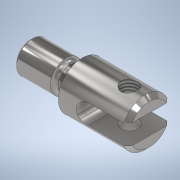
# Autodesk Inventor part: Part11.End Fork
Saved by Autodesk Inventor 2022.2 (Build 262287010, 287A)
## iProperties
Created: 2022-12-06
Part Number: Part11.End Fork
Material: Steel, Carbon
Document SubType Name: Modeling
Designer: User
Density: 7.85 g/cm^3
Appearance: Steel - Polished
Author: User
Autodesk Inventor part; units mm, degrees
ref_plane "YZ Plane" through (0, 0, 0) normal (1, 0, 0) x (0, 1, 0)
ref_plane "XY Plane" through (0, 0, 0) normal (0, 0, 1) x (1, 0, 0)
sketch "Sketch1" plane through (0, 0, 0) normal (1, 0, 0) x (0, 1, 0)
  circle A0 centre (0, 0) radius 12
  dimension "d0" = 24
  constraints: 1 centre point, 1 coincident
  measures "d0" diameter of A0
extrude "Extrusion1" add sketch "Sketch1" along normal blind 34
chamfer "Chamfer1" distance 2 angle 45 1 edges at (34, -12, 0)
sketch "Sketch2" plane through (0, 0, 0) normal (0, 0, 1) x (1, 0, 0)
  line L0 (0, -12) -> (0, 12) construction
  line L1 (32, -12) -> (32, 12) construction
  line L2 (0, 0) -> (32, 0) construction
  line L3 (14, 5) -> (34, 5)
  line L4 (34, -5) -> (14, -5)
  line L5 (34, 10) -> (34, -10) projected
  arc A0 (14, 5) -> (14, -5) centre (14, 0) ccw
  dimension "d8" = 10
  dimension "d9" = 5
  constraints: 6 end point, 2 point on circle, 2 tangent, 1 centre point, 1 horizontal, 1 midpoint, 1 parallel
  measures "d8" distance between parallel lines of L4 L3
  measures "d9" radius of A0
extrude "Extrusion2" cut sketch "Sketch2" along normal through all both and the other way through all
sketch "Sketch5" plane through (0, 0, 0) normal (1, 0, 0) x (0, 1, 0)
  circle A0 centre (0, 0) radius 12 construction
  circle A1 centre (0, 0) radius 6
  dimension "d27" = 12
  constraints: 1 centre point, 1 coincident
  measures "d27" diameter of A1
extrude "Extrusion3" add sketch "Sketch5" against normal blind 8
sketch "Sketch6" plane through (-8, 0, 0) normal (-1, 0, 0) x (0, 0, 1)
  circle A0 centre (0, 0) radius 6 projected
  circle A1 centre (0, 0) radius 8
  dimension "d30" = 16
  constraints: 1 centre point, 1 coincident
  measures "d30" diameter of A1
extrude "Extrusion4" add sketch "Sketch6" along normal blind 18 contours A0 | A1
fillet "Fillet1" radius 2 2 edges at (0, -6, 0) (-8, -6, 0)
chamfer "Chamfer2" distance 1 angle 45 1 edges at (-26, 0, -8)
sketch "Sketch7" plane through (-26, 0, 0) normal (-1, 0, 0) x (0, 0, 1)
  circle A0 centre (0, 0) radius 8 projected
  constraints: 1 coincident
hole "Hole3" at (-26, 0, 0) direction (1, 0, 0) diameter 6.647 depth 22.2 tip angle 118 thread size "M8x1.25" class "6H" standard "ISO Metric profile"
ref_plane "Work Plane1" through (0, 12, 0) normal (0, 1, 0) x (-1, 0, 0)
sketch "Sketch9" plane through (0, 12, 0) normal (0, 1, 0) x (-1, 0, 0)
  line L0 (0, 12) -> (0, -12) construction
  line L1 (-32, 10.9087) -> (-14, 10.9087) construction
  line L2 (-14, 10.9087) -> (-32, 10.9087) construction
  line L3 (-32, -10.9087) -> (-32, 10.9087) construction
  line L4 (-32, -10.9087) -> (-14, -10.9087) construction
  line L5 (-14, -10.9087) -> (-32, -10.9087) construction
  line L6 (-32, 10.9087) -> (-32, -10.9087) construction
  line L7 (-34, -8.6603) -> (-34, 8.6603) construction
  point P0 (0, 0)
  point P1 (-24, 0)
  point P2 (-34, 0)
  dimension "d52" = 10
  constraints: 1 horizontal alignment, 1 midpoint
  measures "d52" distance from line of L7 point (-24, 0)
hole "Hole5" at (24, 12, 0) direction (0, -1, 0) diameter 8.376 depth 27.3 tip angle 118 thread size "M10x1.5" class "6H" standard "ISO Metric profile"
body "Solid1"
